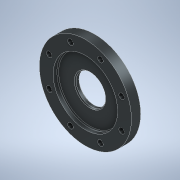
# Autodesk Inventor part: Крышка перегородки12
Saved by Autodesk Inventor 2021 (Build 250183000, 183)
## iProperties
Created: 2020-11-17
Part Number: Крышка перегородки12
Material: Чугун, серый
Document SubType Name: Modeling
Designer: Тимоха
Density: 7.15 g/cm^3
Appearance: Чугун серый
Mass: 3029.23 g
Surface Area: 787.554 cm^2
Volume: 423.669 cm^3
Author: Тимоха
Autodesk Inventor part; units mm, degrees
ref_plane "YZ Plane" through (0, 0, 0) normal (1, 0, 0) x (0, 1, 0)
ref_plane "XZ Plane" through (0, 0, 0) normal (0, 1, 0) x (-1, 0, 0)
ref_plane "XY Plane" through (0, 0, 0) normal (0, 0, 1) x (1, 0, 0)
sketch "Эскиз1" plane through (0, 0, 0) normal (0, 0, 1) x (1, 0, 0)
  circle A0 centre (0, 0) radius 32
  circle A1 centre (0, 0) radius 100
  dimension "d0" = 64
  dimension "d1" = 200
  constraints: 2 centre point, 2 coincident
  measures "d0" diameter of A0
  measures "d1" diameter of A1
extrude "Выдавливание1" add sketch "Эскиз1" along normal blind 10
sketch "Эскиз2" plane through (0, 0, 10) normal (0, 0, 1) x (1, 0, 0)
  circle A0 centre (0, 0) radius 100 projected
  circle A1 centre (0, 0) radius 70
  dimension "d4" = 140
  constraints: 1 centre point, 1 coincident
  measures "d4" diameter of A1
extrude "Выдавливание2" add sketch "Эскиз2" along normal blind 10
fillet "Сопряжение1" radius 2 1 edges at (-70, 0, 10)
chamfer "Фаска1" distance 2 angle 45 2 edges at (-32, 0, 10) (-32, 0, 0)
sketch "Эскиз3" plane through (0, 0, 0) normal (0, 0, -1) x (-1, 0, 0)
  circle A0 centre (0, 0) radius 100 projected
  line L0 (0, 0) -> (78.5298, 32.5281)
  line L1 (140, 0) -> (-140, 0) projected
  dimension "d11" = 85
  dimension "d12" = 22.5
  constraints: 2 end point
  measures "d11" distance of L0.start L0.end
  measures "d12" angle of L1 L0
hole "Отверстие1" at (-78.5298, 32.5281, 0) direction (0, 0, 1) diameter 12 end through all
pattern_circular "Круговой массив1" count 8 over 360 about axis through (0, 0, 1) along (0, 0, 1) of "Отверстие1"
